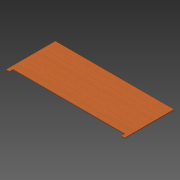
# Autodesk Inventor part: top-plate
Saved by Autodesk Inventor 2013 (Build 170138000, 138)
## iProperties
Created: 2013-05-01
Part Number: top-plate
Material: Wood (Cherry)
Document SubType Name: Modeling
Designer: Chris
Density: 0.5 g/cm^3
Mass: 5308.38 g
Surface Area: 17259.6 cm^2
Volume: 10616.8 cm^3
Author: Chris
Autodesk Inventor part; units mm, degrees
ref_plane "YZ Plane" through (0, 0, 0) normal (1, 0, 0) x (0, 1, 0)
ref_plane "XZ Plane" through (0, 0, 0) normal (0, 1, 0) x (-1, 0, 0)
ref_plane "XY Plane" through (0, 0, 0) normal (0, 0, 1) x (1, 0, 0)
sketch "Sketch1" plane through (0, 0, 0) normal (0, 1, 0) x (-1, 0, 0)
  line L0 (0, 0) -> (1473.2, 0)
  line L1 (1473.2, 0) -> (1473.2, 609.6)
  line L2 (1473.2, 609.6) -> (0, 609.6)
  line L3 (0, 609.6) -> (0, 0)
  line L4 (1435.1, 609.6) -> (1435.1, 565.15)
  line L5 (1435.1, 565.15) -> (38.1, 565.15)
  line L6 (38.1, 565.15) -> (38.1, 609.6)
  dimension "d0" = 1473.2
  dimension "d1" = 609.6
  dimension "d4" = 44.45
  dimension "d10" = 38.1
  dimension "d11" = 38.1
  constraints: 14 end point, 4 parallel, 2 horizontal, 2 perpendicular, 2 point on line
  measures "d0" distance of L2.end L1.end
  measures "d1" distance of L1.end L0.end
  measures "d4" distance of L4.start L4.end
  measures "d10" distance between parallel lines of L3 L6
  measures "d11" distance between parallel lines of L1 L4
extrude "Extrusion2" add sketch "Sketch1" along normal blind 12.7 contours L3 L2 L6 L5 L4 L1 L0
body "Solid2"
